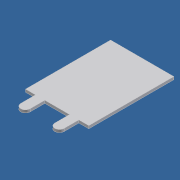
# Autodesk Inventor part: M202830TX-switch
Saved by Autodesk Inventor 2014 (Build 180170000, 170)
## iProperties
Category: PARTsolutions
Created: 2013-12-29
Part Number: M202830TX-switch
Catalog Web Link: www.cadenas.de
Description: Angle Mount Miniature Rockers - Shroud Terminals - Series M - Miniature Rockers
Document SubType Name: Modeling
Designer: PARTsolutions
Material: Generic
Density: 1 g/cm^3
Appearance: RGB(192,192,192)
NB: M202830TX-switch
NN: Angle Mount Miniature Rockers - Shroud Terminals
NT: Series M - Miniature Rockers
NBSYN: $PN.-switch
LINA: M202830TX-switch
PN: M202830TX
SRS: M20
PLS: 2
CRCTSALG: '2','2 - ON/NONE/ON','3','3 - ON/OFF/ON','5','5 - ON/NONE/(ON)','8','8 - (ON)/OFF/(ON)','9','9 - ON/OFF/(ON)','4', '4 - ON/ON/ON','6','6 - (ON)/ON/(ON)','7','7 - ON/ON/(ON)'
CRCTS: 8
FRMALG: 'TX', 'TX - Narrow Frame for Small Actuator', 'TZ'  , 'TZ - Wide Frame for Large Actuator'
FRM: TX
TRMNLSALG: '30', '30 - .150" (3.81mm) Right Angle PC (1-3 Pole)', '32'  , '32 -  Right Angle PCB (1 Pole & 0.4VA Rating Only', '40'  , '40 - .150" (3.81mm) Vertical PC (1-4 Pole)', '45'  , '45 - .100" (2.54mm) Vertical PC (1-4 Pole)'
TRMNLS: 30
WIDTH: 0.512
HEIGHT: 0.388
LENGTH: 0.500
A: 0.150
TRMNLNOH: 2.000
TRMNLOV: 3.000
LTRMNL: 0.031
POS: 0.075
POS2: 0.185
POS3: 0.150
D: 0.075
HOLES: 0.185
WH: 0.15000
D1: 0.00000
D2: 0.07500
KT: DUMMY
SUPPLIER: NKKSWITCHES
ARTICLENO: M202830TX-switch
BOMINFO: M202830TX-switch
CREATOR: CADENAS GmbH
PSOL_IDENT_0: {$CADENAS_DATA\23d-libs\nkkswitches\toggle\m\parts\m_ang_t_shroudterm.prj},236 {VTYP=3D},{NB=M202830
PSOL_IDENT_1: TX-switch},{LINA=M202830TX-switch},{NN=Angle Mount Miniature Rockers - Shroud Terminals},{DATE=28.05
PSOL_IDENT_2: .2007 07:27:48},{GEOMDATE=28.05.2007 00:00:00},{VERSION=},{LINEID=10},{LINESUBID=-1},{WBVAR=PLS,CRCT
PSOL_IDENT_3: S,FRM,TRMNLS}  {NB=M202830TX-switch},{LINA=M202830TX-switch},{KT=DUMMY},{PN=M202830TX},{SRS=M20},{PL
PSOL_IDENT_4: S=2},{CRCTSALG='2','2 - ON/NONE/ON','3','3 - ON/OFF/ON','5','5 - ON/NONE/(ON)','8','8 - (ON)/OFF/(ON
PSOL_IDENT_5: )','9','9 - ON/OFF/(ON)','4', '4 - ON/ON/ON','6','6 - (ON)/ON/(ON)','7','7 - ON/ON/(ON)'},{CRCTS=8},
PSOL_IDENT_6: {FRMALG='TX', 'TX - Narrow Frame for Small Actuator', 'TZ'  , 'TZ - Wide Frame for Large Actuator'},
PSOL_IDENT_7: {FRM=TX},{TRMNLSALG='30', '30 - .150\" (3.81mm) Right Angle PC (1-3 Pole)', '32'  , '32 -  Right Ang
PSOL_IDENT_8: le PCB (1 Pole & 0.4VA Rating Only', '40'  , '40 - .150\" (3.81mm) Vertical PC (1-4 Pole)', '45'  ,
PSOL_IDENT_9: '45 - .100\" (2.54mm) Vertical PC (1-4 Pole)'},{TRMNLS=30},{WIDTH=0.512},{HEIGHT=0.3877},{LENGTH=0.5
PSOL_IDENT_10: },{A=0.15},{TRMNLNOH=2},{TRMNLOV=3},{LTRMNL=0.031},{POS=0.075},{POS2=0.185},{POS3=0.15},{D=0.075},{H
PSOL_IDENT_11: OLES=0.185},{WH=0.15000},{D1=0.00000},{D2=0.07500}
Title: M202830TX-switch
Author: Cadenas PARTsolutions
Comments: Series M - Miniature Rockers
Autodesk Inventor part; units mm, degrees
sketch "Sketch_1" plane through (0, 0, 0) normal (0, 1, 0) x (-1, 0, 0)
  line L0 (4.7244, 6.35) -> (3.2385, 6.35)
  line L1 (3.2385, 6.35) -> (3.2385, 8.5471)
  arc A0 (3.2385, 8.5471) -> (1.8415, 8.5471) centre (2.54, 8.5471) ccw
  line L2 (1.8415, 8.5471) -> (1.8415, 6.35)
  line L3 (1.8415, 6.35) -> (-1.8415, 6.35)
  line L4 (-1.8415, 6.35) -> (-1.8415, 8.5471)
  arc A1 (-1.8415, 8.5471) -> (-3.2385, 8.5471) centre (-2.54, 8.5471) ccw
  line L5 (-3.2385, 8.5471) -> (-3.2385, 6.35)
  line L6 (-3.2385, 6.35) -> (-4.7244, 6.35)
  line L7 (-4.7244, 6.35) -> (-4.7244, -6.35)
  line L8 (-4.7244, -6.35) -> (4.7244, -6.35)
  line L9 (4.7244, -6.35) -> (4.7244, 6.35)
  constraints: 20 end point, 4 point on circle, 2 centre point
extrude "Extrusion1" add sketch "Sketch_1" along normal blind 0.4064
ref_plane "shtrmnl_XY" through (0, 0, 0) normal (0, 1, 0) x (1, 0, 0)
ref_plane "shtrmnl_YZ" through (0, 0, 0) normal (1, 0, 0) x (0, 0, -1)
ref_plane "shtrmnl_ZX" through (0, 0, 0) normal (0, 0, -1) x (0, 1, 0)
body "Solid1"
